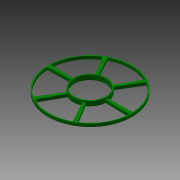
# Autodesk Inventor part: Wheel-190D-Join
Saved by Autodesk Inventor 2014 SP1 (Build 180222100, 222)
## iProperties
Created: 2017-01-25
Part Number: Wheel-190D-Join
Material: Generic
Document SubType Name: Modeling
Designer: danielsikar
Density: 1 g/cm^3
Appearance: Dark Green
Author: danielsikar
Autodesk Inventor part; units mm, degrees
ref_plane "Work Plane1" through (6.7321, 7.6603, 6.5) normal (0, 0, -1) x (-1, 0, 0)
ref_plane "Work Plane2" through (-91.9966, 5.6978, 0) normal (0, 0, 1) x (1, 0, 0)
sketch "Sketch2" plane through (6.7321, 7.6603, 6.5) normal (0, 0, -1) x (-1, 0, 0)
  arc A0 (-24.9048, 4.5792) -> (-24.9048, -0.5792) centre (10, 2) ccw projected
  line L0 (-24.9048, 4.5792) -> (-78.8985, 5.8348) projected
  spline S0 degree 3 poles (-81.8209, 7.9406) (-81.8261, 7.8611) (-81.8206, 7.7825) (-81.7897, 7.6241) (-81.7641, 7.5464) (-81.6606, 7.31) (-81.5548, 7.1589) (-81.2411, 6.7962) (-80.9721, 6.571) (-80.3946, 6.2158) (-80.1028, 6.0812) (-79.5089, 5.8959) (-79.2045, 5.842) (-78.8985, 5.8348) knots 0 0 0 0 0.0239 0.0239 0.048426 0.048426 0.101393 0.101393 0.192693 0.192693 0.27175 0.27175 0.348512 0.348512 0.348512 0.348512 projected
  arc A1 (-41.0552, 78.5489) -> (-81.8209, 7.9406) centre (10, 2) ccw projected
  spline S1 degree 3 poles (-37.7703, 77.0709) (-37.9792, 77.4141) (-38.2566, 77.7144) (-38.9885, 78.2905) (-39.4509, 78.5125) (-40.0652, 78.6833) (-40.2919, 78.7218) (-40.6062, 78.7092) (-40.7048, 78.6952) (-40.8909, 78.6405) (-40.9762, 78.6017) (-41.0552, 78.5489) knots 0 0 0 0 0.120544 0.120544 0.279074 0.279074 0.360181 0.360181 0.397351 0.397351 0.43301 0.43301 0.43301 0.43301 projected
  line L1 (-9.6861, 30.9389) -> (-37.7703, 77.0709) projected
  arc A2 (-5.2188, 33.5181) -> (-9.6861, 30.9389) centre (10, 2) ccw projected
  line L2 (-5.2188, 33.5181) -> (-31.1282, 80.9057) projected
  spline S2 degree 3 poles (-30.7657, 84.4896) (-30.8731, 84.4365) (-30.9658, 84.364) (-31.1483, 84.1647) (-31.2278, 84.0319) (-31.3942, 83.6678) (-31.4659, 83.3963) (-31.5524, 82.7609) (-31.5541, 82.3658) (-31.4249, 81.594) (-31.3074, 81.2336) (-31.1282, 80.9057) knots 0 0 0 0 0.035944 0.035944 0.08118 0.08118 0.156549 0.156549 0.248753 0.248753 0.333217 0.333217 0.333217 0.333217 projected
  arc A3 (50.7657, 84.4896) -> (-30.7657, 84.4896) centre (10, 2) ccw projected
  spline S3 degree 3 poles (51.1282, 80.9057) (51.3209, 81.2583) (51.4423, 81.6486) (51.5753, 82.5706) (51.5364, 83.082) (51.3771, 83.6993) (51.2971, 83.9149) (51.129, 84.1809) (51.0676, 84.2592) (50.9272, 84.393) (50.8509, 84.4475) (50.7657, 84.4896) knots 0 0 0 0 0.120544 0.120544 0.279074 0.279074 0.360181 0.360181 0.397351 0.397351 0.43301 0.43301 0.43301 0.43301 projected
  line L3 (25.2188, 33.5181) -> (51.1282, 80.9057) projected
  arc A4 (29.6861, 30.9389) -> (25.2188, 33.5181) centre (10, 2) ccw projected
  line L4 (29.6861, 30.9389) -> (57.7703, 77.0709) projected
  spline S4 degree 3 poles (61.0552, 78.5489) (60.9555, 78.6154) (60.8464, 78.6595) (60.5826, 78.7178) (60.4278, 78.7203) (60.0293, 78.6823) (59.7583, 78.6087) (59.1648, 78.3659) (58.8217, 78.1698) (58.218, 77.672) (57.9646, 77.39) (57.7703, 77.0709) knots 0 0 0 0 0.035944 0.035944 0.08118 0.08118 0.156549 0.156549 0.248753 0.248753 0.333217 0.333217 0.333217 0.333217 projected
  arc A5 (101.8209, 7.9406) -> (61.0552, 78.5489) centre (10, 2) ccw projected
  spline S5 degree 3 poles (98.8985, 5.8348) (99.3002, 5.8442) (99.6989, 5.9342) (100.5638, 6.28) (100.9872, 6.5694) (101.4422, 7.0161) (101.5889, 7.1931) (101.7352, 7.4717) (101.7724, 7.564) (101.8181, 7.7525) (101.8271, 7.8458) (101.8209, 7.9406) knots 0 0 0 0 0.120544 0.120544 0.279074 0.279074 0.360181 0.360181 0.397351 0.397351 0.43301 0.43301 0.43301 0.43301 projected
  line L5 (44.9048, 4.5792) -> (98.8985, 5.8348) projected
  arc A6 (44.9048, -0.5792) -> (44.9048, 4.5792) centre (10, 2) ccw projected
  line L6 (44.9048, -0.5792) -> (98.8985, -1.8348) projected
  spline S6 degree 3 poles (101.8209, -3.9406) (101.8287, -3.8211) (101.8123, -3.7046) (101.7308, -3.4469) (101.6557, -3.3116) (101.4235, -2.9855) (101.2242, -2.7876) (100.7172, -2.395) (100.3759, -2.196) (99.6429, -1.922) (99.272, -1.8435) (98.8985, -1.8348) knots 0 0 0 0 0.035944 0.035944 0.08118 0.08118 0.156549 0.156549 0.248753 0.248753 0.333217 0.333217 0.333217 0.333217 projected
  arc A7 (61.0552, -74.5489) -> (101.8209, -3.9406) centre (10, 2) ccw projected
  spline S7 degree 3 poles (57.7703, -73.0709) (57.9792, -73.4141) (58.2566, -73.7144) (58.9885, -74.2905) (59.4509, -74.5125) (60.0652, -74.6833) (60.2919, -74.7218) (60.6062, -74.7092) (60.7048, -74.6952) (60.8909, -74.6405) (60.9762, -74.6017) (61.0552, -74.5489) knots 0 0 0 0 0.120544 0.120544 0.279074 0.279074 0.360181 0.360181 0.397351 0.397351 0.43301 0.43301 0.43301 0.43301 projected
  line L7 (29.6861, -26.9389) -> (57.7703, -73.0709) projected
  arc A8 (25.2188, -29.5181) -> (29.6861, -26.9389) centre (10, 2) ccw projected
  line L8 (25.2188, -29.5181) -> (51.1282, -76.9057) projected
  spline S8 degree 3 poles (50.7657, -80.4896) (50.8731, -80.4365) (50.9658, -80.364) (51.1483, -80.1647) (51.2278, -80.0319) (51.3942, -79.6678) (51.4659, -79.3963) (51.5524, -78.7609) (51.5541, -78.3658) (51.4249, -77.594) (51.3074, -77.2336) (51.1282, -76.9057) knots 0 0 0 0 0.035944 0.035944 0.08118 0.08118 0.156549 0.156549 0.248753 0.248753 0.333217 0.333217 0.333217 0.333217 projected
  arc A9 (-30.7657, -80.4896) -> (50.7657, -80.4896) centre (10, 2) ccw projected
  spline S9 degree 3 poles (-31.1282, -76.9057) (-31.3209, -77.2583) (-31.4423, -77.6486) (-31.5753, -78.5706) (-31.5364, -79.082) (-31.3771, -79.6993) (-31.2971, -79.9149) (-31.129, -80.1809) (-31.0676, -80.2592) (-30.9272, -80.393) (-30.8509, -80.4475) (-30.7657, -80.4896) knots 0 0 0 0 0.120544 0.120544 0.279074 0.279074 0.360181 0.360181 0.397351 0.397351 0.43301 0.43301 0.43301 0.43301 projected
  line L9 (-5.2188, -29.5181) -> (-31.1282, -76.9057) projected
  arc A10 (-9.6861, -26.9389) -> (-5.2188, -29.5181) centre (10, 2) ccw projected
  line L10 (-9.6861, -26.9389) -> (-37.7703, -73.0709) projected
  spline S10 degree 3 poles (-41.0552, -74.5489) (-40.9555, -74.6154) (-40.8464, -74.6595) (-40.5826, -74.7178) (-40.4278, -74.7203) (-40.0293, -74.6823) (-39.7583, -74.6087) (-39.1648, -74.3659) (-38.8217, -74.1698) (-38.218, -73.672) (-37.9646, -73.39) (-37.7703, -73.0709) knots 0 0 0 0 0.035944 0.035944 0.08118 0.08118 0.156549 0.156549 0.248753 0.248753 0.333217 0.333217 0.333217 0.333217 projected
  arc A11 (-81.8209, -3.9406) -> (-41.0552, -74.5489) centre (10, 2) ccw projected
  spline S11 degree 3 poles (-78.8985, -1.8348) (-79.3002, -1.8442) (-79.6989, -1.9342) (-80.5638, -2.28) (-80.9872, -2.5694) (-81.4422, -3.0161) (-81.5889, -3.1931) (-81.7352, -3.4717) (-81.7724, -3.564) (-81.8181, -3.7525) (-81.8271, -3.8458) (-81.8209, -3.9406) knots 0 0 0 0 0.120544 0.120544 0.279074 0.279074 0.360181 0.360181 0.397351 0.397351 0.43301 0.43301 0.43301 0.43301 projected
  line L11 (-24.9048, -0.5792) -> (-78.8985, -1.8348) projected
  line L12 (-84.2597, 5.9595) -> (-84.3419, 2.4266) projected
  arc A12 (-84.3419, 2.4266) -> (-40.5589, -77.6516) centre (10, 2) ccw projected
  line L13 (-40.5589, -77.6516) -> (-33.7892, -81.7728) projected
  line L14 (-33.7008, -81.6111) -> (-33.7892, -81.7728) projected
  arc A13 (-33.7008, -81.6111) -> (53.7008, -81.6111) centre (10, 2) ccw projected
  line L15 (53.7008, -81.6111) -> (60.6548, -77.809) projected
  line L16 (60.5589, -77.6516) -> (60.6548, -77.809) projected
  arc A14 (60.5589, -77.6516) -> (104.2597, -1.9595) centre (10, 2) ccw projected
  line L17 (104.2597, -1.9595) -> (104.444, 5.9638) projected
  line L18 (104.2597, 5.9595) -> (104.444, 5.9638) projected
  arc A15 (104.2597, 5.9595) -> (60.5589, 81.6516) centre (10, 2) ccw projected
  line L19 (60.5589, 81.6516) -> (53.7892, 85.7728) projected
  line L20 (53.7008, 85.6111) -> (53.7892, 85.7728) projected
  arc A16 (53.7008, 85.6111) -> (-33.7008, 85.6111) centre (10, 2) ccw projected
  line L21 (-33.7008, 85.6111) -> (-40.6548, 81.809) projected
  line L22 (-40.5589, 81.6516) -> (-40.6548, 81.809) projected
  arc A17 (-40.5589, 81.6516) -> (-84.2597, 5.9595) centre (10, 2) ccw projected
  point P0 (6.7321, -7.6603)
extrude "Extrusion1" add sketch "Sketch2" along normal up to surface (6.5 mm away)
ref_plane "Work Plane3" through (-3.2679, 9.6603, 1.5) normal (0, 0, 1) x (1, 0, 0)
sketch "Sketch3" plane through (-3.2679, 9.6603, 1.5) normal (0, 0, 1) x (1, 0, 0)
  circle A0 centre (0, 0) radius 35
  circle A1 centre (0, 0) radius 37.5
  point P0 (3.2679, -9.6603)
  dimension "d2" = 70
  dimension "d3" = 75
  constraints: 2 centre point, 1 coincident
  measures "d2" diameter of A0
  measures "d3" diameter of A1
ref_plane "Work Plane4" through (11.9508, 38.5991, 10.5) normal (0, 0, 1) x (1, 0, 0)
extrude "Extrusion2" add sketch "Sketch3" along normal up to surface (9 mm away)
sketch "Sketch4" plane through (-3.2679, 9.6603, 1.5) normal (0, 0, -1) x (-1, 0, 0)
  arc A0 (-16.4195, -33.7142) -> (16.4195, -33.7142) centre (0, 0) ccw projected
  circle A1 centre (0, 0) radius 35
  circle A2 centre (0, 0) radius 37.5
  point P0 (-3.2679, -9.6603)
  dimension "d6" = 70
  dimension "d7" = 75
  constraints: 2 centre point, 2 coincident
  measures "d6" diameter of A1
  measures "d7" diameter of A2
extrude "Extrusion3" add sketch "Sketch4" along normal up to surface (1.5 mm away)
body "Solid1"
